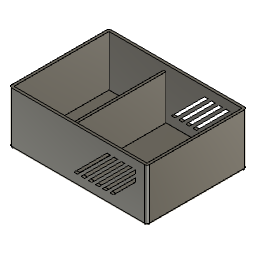
case (Autodesk Fusion 360 design; units mm, degrees)
Autodesk Fusion 360 part; units mm, degrees
sketch "Skizze1" plane through (0, 0, 0) normal (0, 0, 1) x (1, 0, 0)
  line L0 (0, 0) -> (105, 0)
  line L1 (105, 0) -> (105, 75)
  line L2 (105, 75) -> (0, 75)
  line L3 (0, 75) -> (0, 0)
  line L4 (0, 40) -> (43, 40) construction
  line L5 (43, 75) -> (45, 75)
  line L6 (45, 75) -> (45, 0)
  line L7 (45, 0) -> (43, 0)
  line L8 (43, 0) -> (43, 75)
  dimension "d1" = 105
  dimension "d2" = 75
  dimension "d7" = 43
  dimension "d8" = 2
  dimension "d9" = 75
  constraint horizontal L0
  constraint vertical L1
  constraint horizontal L2
  constraint vertical L3
  constraint coincident L0.start L3.end
  constraint coincident L3 L4.start
  constraint perpendicular L3 L4
  constraint horizontal L5
  constraint vertical L6
  constraint horizontal L7
  constraint vertical L8
  constraint coincident L2 L5.start
  measures "d1" distance of L0.start L0.end
  measures "d2" distance of L0.start L2.end
  measures "d7" distance of L4.start L4.end
  measures "d8" distance of L5.start L5.end
  measures "d9" distance of L5.start L7.end
extrude "Extrusion1" add sketch "Skizze1" along normal blind 40
shell "Schale1" thickness 2 outward yes removed faces 1 at (85, 25, 40)
extrude "Extrusion2" add sketch "Skizze1" along normal blind 35 contours L0 L2 L5 L6 L7 L8
fillet "Abrundung1" radius 2 8 edges at (107, -2, 19) (107, 37.5, -2) (52.5, -2, -2) (-2, -2, 19) (107, 77, 19) (-2, 37.5, -2) (-2, 77, 19) (52.5, 77, -2)
sketch "Skizze2" plane through (0, -2, 0) normal (0, -1, 0) x (1, 0, 0)
  line L0 (105, 0) -> (105, 40)
  line L1 (105, 40) -> (0, 40)
  line L2 (0, 40) -> (0, 0)
  line L3 (0, 0) -> (105, 0)
  line L4 (105, 40) -> (45, 40) construction
  line L5 (105, 40) -> (65, 0)
  line L6 (105, 40) -> (161.5685, 40) construction
  line L7 (103.5858, 41.4142) -> (63.5858, 1.4142)
  line L8 (102.1716, 42.8284) -> (62.1716, 2.8284)
  line L9 (100.7574, 44.2426) -> (60.7574, 4.2426)
  line L10 (99.3431, 45.6569) -> (59.3431, 5.6569)
  line L11 (106.4142, 38.5858) -> (66.4142, -1.4142)
  line L12 (107.8284, 37.1716) -> (67.8284, -2.8284)
  line L13 (109.2426, 35.7574) -> (69.2426, -4.2426)
  line L14 (7, 7) -> (98, 7)
  line L15 (98, 7) -> (98, 33)
  line L16 (98, 33) -> (7, 33)
  line L17 (7, 33) -> (7, 7)
  line L18 (90.8579, 40) -> (50.8579, 0)
  line L19 (89.4437, 41.4142) -> (49.4437, 1.4142)
  line L20 (88.0294, 42.8284) -> (48.0294, 2.8284)
  line L21 (86.6152, 44.2426) -> (46.6152, 4.2426)
  dimension "d14" = 60
  dimension "d15" = 135
  dimension "d16" = 2
  dimension "d17" = 4
  dimension "d18" = 6
  dimension "d19" = 8
  dimension "d20" = -2
  dimension "d21" = -4
  dimension "d22" = -6
  dimension "d24" = -7
  dimension "d26" = 2
  dimension "d27" = 4
  dimension "d28" = 6
  constraint coincident L0.end L1.start
  constraint perpendicular L0 L4
  constraint horizontal L6
  constraint coincident L3 L5.end
  constraint coincident L1 L18.start
  constraint coincident L3 L18.end
  measures "d14" distance of L0.end L4.end
  measures "d15" angle of L5 L6
extrude "Extrusion3" cut sketch "Skizze2" against normal blind 110 contours L12 L13 L14 L15 | L5 L11 L14 L15 | L7 L8 L14 L16 | L14 L16 L18 L19 | L9 L10 L14 L16 | L14 L16 L20 L21
